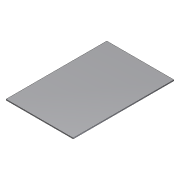
# Autodesk Inventor part: floor
Saved by Autodesk Inventor 2012 (Build 160160000, 160)
## iProperties
Created: 2013-01-12
Part Number: floor
Material: Default
Document SubType Name: Modeling
Designer: JesseK
Mass: 0.453592 g
Surface Area: 17651.6 cm^2
Volume: 21237.6 cm^3
Density: 2.1358e-05 g/cm^3
Author: JesseK
Autodesk Inventor part; units mm, degrees
ref_plane "YZ Plane" through (0, 0, 0) normal (1, 0, 0) x (0, 1, 0)
ref_plane "XZ Plane" through (0, 0, 0) normal (0, 1, 0) x (-1, 0, 0)
ref_plane "XY Plane" through (0, 0, 0) normal (0, 0, 1) x (1, 0, 0)
sketch "Sketch2" plane through (0, 0, 0) normal (0, 1, 0) x (-1, 0, 0)
  line L0 (0, 0) -> (1828.8, 0)
  line L1 (1828.8, 0) -> (1828.8, 2743.2)
  line L2 (1828.8, 2743.2) -> (0, 2743.2)
  line L3 (0, 2743.2) -> (0, 0)
  dimension "d0" = 2743.2
  dimension "d1" = 1828.8
  constraints: 8 end point, 2 parallel, 1 horizontal, 1 perpendicular
  measures "d0" distance of L2.end L0.start
  measures "d1" distance of L0.start L0.end
extrude "Extrusion1" add sketch "Sketch2" along normal blind 25.4
body "Solid1"
